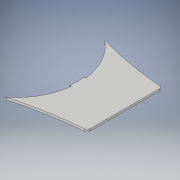
# Autodesk Inventor part: headset cover
Saved by Autodesk Inventor 2018 (Build 220112000, 112)
## iProperties
Created: 2020-07-06
Part Number: headset cover
Material: Generic
Document SubType Name: Modeling
Designer: maqur
Density: 1 g/cm^3
Appearance: Default
Author: maqur
Autodesk Inventor part; units mm, degrees
ref_plane "YZ Plane" through (0, 0, 0) normal (1, 0, 0) x (0, 1, 0)
ref_plane "XZ Plane" through (0, 0, 0) normal (0, 1, 0) x (-1, 0, 0)
ref_plane "XY Plane" through (0, 0, 0) normal (0, 0, 1) x (1, 0, 0)
sketch "Sketch1" plane through (0, 0, 0) normal (0, 1, 0) x (-1, 0, 0)
  arc A0 (5.267, 59.2831) -> (5.267, 39.6662) centre (89.2034, 49.4746) ccw
  spline S0 degree 3 poles (5.1685, 59.2746) (5.2015, 59.2746) (5.2345, 59.2774) (5.267, 59.2831) knots -0.075945 -0.075945 -0.075945 -0.075945 -0.065858 -0.065858 -0.065858 -0.065858
  line L0 (3.4, 59.2746) -> (5.1685, 59.2746)
  arc A1 (2.9135, 59.8229) -> (3.4, 59.2746) centre (3.4, 59.7645) ccw
  arc A2 (34.9269, 117.3502) -> (2.9135, 59.8229) centre (89.2034, 49.4746) ccw
  arc A3 (-57.0396, 100.9066) -> (34.9269, 117.3502) centre (-97.4277, 592.1892) ccw
  arc A4 (-57.0396, 100.9066) -> (-60.4248, 97.2317) centre (-56.7375, 97.2317) ccw
  line L1 (-60.4248, 1.7175) -> (-60.4248, 97.2317)
  arc A5 (-60.4248, 1.7175) -> (-57.0396, -1.9573) centre (-56.7375, 1.7175) ccw
  arc A6 (34.9269, -18.4009) -> (-57.0396, -1.9573) centre (-97.4277, -493.24) ccw
  arc A7 (2.9135, 39.1264) -> (34.9269, -18.4009) centre (89.2034, 49.4746) ccw
  arc A8 (3.4, 39.6746) -> (2.9135, 39.1264) centre (3.4, 39.1847) ccw
  line L2 (3.4, 39.6746) -> (5.1685, 39.6746)
  spline S1 degree 3 poles (5.267, 39.6662) (5.2345, 39.6718) (5.2015, 39.6746) (5.1685, 39.6746) knots -0.010125 -0.010125 -0.010125 -0.010125 0 0 0 0
  point P0 (0, 0)
  point P1 (-1.1347, 1.9446)
  constraints: 18 point on circle, 9 centre point, 6 end point, 6 other
extrude "Extrusion1" add sketch "Sketch1" along normal blind 3
body "Solid1"
